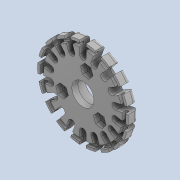
# Autodesk Inventor part: PartA
Saved by Autodesk Inventor 2020.4 (Build 244396000, 396)
## iProperties
Created: 2020-04-29
Part Number: PartA
Material: ABS Plastic
Document SubType Name: Modeling
Designer: Acer
Density: 1.06 g/cm^3
Appearance: Smooth - Black
Author: Acer
Autodesk Inventor part; units mm, degrees
ref_plane "YZ Plane" through (0, 0, 0) normal (1, 0, 0) x (0, 1, 0)
ref_plane "XZ Plane" through (0, 0, 0) normal (0, 1, 0) x (-1, 0, 0)
ref_plane "XY Plane" through (0, 0, 0) normal (0, 0, 1) x (1, 0, 0)
sketch "Sketch1" plane through (0, 0, 0) normal (0, 0, 1) x (1, 0, 0)
  circle A0 centre (0, 0) radius 22.5
  dimension "d0" = 45
  constraints: 1 centre point, 1 coincident
  measures "d0" diameter of A0
extrude "PartA Base" add sketch "Sketch1" along normal blind 7
sketch "Sketch2" plane through (0, 0, 0) normal (0, 0, -1) x (-1, 0, 0)
  circle A0 centre (0, 0) radius 13.5
  circle A1 centre (0, 0) radius 22.5 projected
  dimension "d3" = 27
  constraints: 1 centre point, 1 coincident
  measures "d3" diameter of A0
extrude "Shaft Entrance" cut sketch "Sketch2" against normal blind 2
sketch "Sketch3" plane through (0, 0, 7) normal (0, 0, 1) x (1, 0, 0)
  line L0 (0, 22.95) -> (0, 16.25) construction
  line L1 (-1.6, 22.95) -> (-1.6, 16.25)
  line L2 (1.6, 16.25) -> (1.6, 22.95)
  arc A0 (1.6, 22.95) -> (-1.6, 22.95) centre (0, 22.95) ccw
  arc A1 (-1.6, 16.25) -> (1.6, 16.25) centre (0, 16.25) ccw
  line L3 (0, 22.95) -> (6.7, 22.95) construction
  line L4 (-4.0543, 15.8172) -> (-6.3459, 22.1132)
  arc A2 (-7.0613, 14.7228) -> (-4.0543, 15.8172) centre (-5.5578, 15.27) ccw
  line L5 (-7.8494, 21.5659) -> (-5.5578, 15.27) construction
  arc A3 (-6.3459, 22.1132) -> (-9.3529, 21.0187) centre (-7.8494, 21.5659) ccw
  line L6 (-9.3529, 21.0187) -> (-7.0613, 14.7228)
  line L7 (-7.8494, 21.5659) -> (-1.5534, 23.8575) construction
  line L8 (-9.2196, 13.4767) -> (-13.5263, 18.6092)
  arc A4 (-11.671, 11.4198) -> (-9.2196, 13.4767) centre (-10.4453, 12.4482) ccw
  line L9 (-14.752, 17.5807) -> (-10.4453, 12.4482) construction
  arc A5 (-13.5263, 18.6092) -> (-15.9776, 16.5523) centre (-14.752, 17.5807) ccw
  line L10 (-15.9776, 16.5523) -> (-11.671, 11.4198)
  line L11 (-14.752, 17.5807) -> (-9.6195, 21.8874) construction
  line L12 (-13.2729, 9.5106) -> (-19.0753, 12.8606)
  arc A6 (-14.8729, 6.7394) -> (-13.2729, 9.5106) centre (-14.0729, 8.125) ccw
  line L13 (-19.8753, 11.475) -> (-14.0729, 8.125) construction
  arc A7 (-19.0753, 12.8606) -> (-20.6753, 10.0894) centre (-19.8753, 11.475) ccw
  line L14 (-20.6753, 10.0894) -> (-14.8729, 6.7394)
  line L15 (-19.8753, 11.475) -> (-16.5253, 17.2774) construction
  line L16 (-15.7253, 4.3975) -> (-22.3235, 5.5609)
  arc A8 (-16.281, 1.2461) -> (-15.7253, 4.3975) centre (-16.0031, 2.8218) ccw
  line L17 (-22.6013, 3.9852) -> (-16.0031, 2.8218) construction
  arc A9 (-22.3235, 5.5609) -> (-22.8792, 2.4095) centre (-22.6013, 3.9852) ccw
  line L18 (-22.8792, 2.4095) -> (-16.281, 1.2461)
  line L19 (-22.6013, 3.9852) -> (-21.4379, 10.5834) construction
  line L20 (-16.281, -1.2461) -> (-22.8792, -2.4095)
  arc A10 (-15.7253, -4.3975) -> (-16.281, -1.2461) centre (-16.0031, -2.8218) ccw
  line L21 (-22.6013, -3.9852) -> (-16.0031, -2.8218) construction
  arc A11 (-22.8792, -2.4095) -> (-22.3235, -5.5609) centre (-22.6013, -3.9852) ccw
  line L22 (-22.3235, -5.5609) -> (-15.7253, -4.3975)
  line L23 (-22.6013, -3.9852) -> (-23.7648, 2.613) construction
  line L24 (-14.8729, -6.7394) -> (-20.6753, -10.0894)
  arc A12 (-13.2729, -9.5106) -> (-14.8729, -6.7394) centre (-14.0729, -8.125) ccw
  line L25 (-19.8753, -11.475) -> (-14.0729, -8.125) construction
  arc A13 (-20.6753, -10.0894) -> (-19.0753, -12.8606) centre (-19.8753, -11.475) ccw
  line L26 (-19.0753, -12.8606) -> (-13.2729, -9.5106)
  line L27 (-19.8753, -11.475) -> (-23.2253, -5.6726) construction
  line L28 (-11.671, -11.4198) -> (-15.9776, -16.5523)
  arc A14 (-9.2196, -13.4767) -> (-11.671, -11.4198) centre (-10.4453, -12.4482) ccw
  line L29 (-14.752, -17.5807) -> (-10.4453, -12.4482) construction
  arc A15 (-15.9776, -16.5523) -> (-13.5263, -18.6092) centre (-14.752, -17.5807) ccw
  line L30 (-13.5263, -18.6092) -> (-9.2196, -13.4767)
  line L31 (-14.752, -17.5807) -> (-19.8845, -13.274) construction
  line L32 (-7.0613, -14.7228) -> (-9.3529, -21.0187)
  arc A16 (-4.0543, -15.8172) -> (-7.0613, -14.7228) centre (-5.5578, -15.27) ccw
  line L33 (-7.8494, -21.5659) -> (-5.5578, -15.27) construction
  arc A17 (-9.3529, -21.0187) -> (-6.3459, -22.1132) centre (-7.8494, -21.5659) ccw
  line L34 (-6.3459, -22.1132) -> (-4.0543, -15.8172)
  line L35 (-7.8494, -21.5659) -> (-14.1453, -19.2744) construction
  line L36 (-1.6, -16.25) -> (-1.6, -22.95)
  arc A18 (1.6, -16.25) -> (-1.6, -16.25) centre (0, -16.25) ccw
  line L37 (0, -22.95) -> (0, -16.25) construction
  arc A19 (-1.6, -22.95) -> (1.6, -22.95) centre (0, -22.95) ccw
  line L38 (1.6, -22.95) -> (1.6, -16.25)
  line L39 (0, -22.95) -> (-6.7, -22.95) construction
  line L40 (4.0543, -15.8172) -> (6.3459, -22.1132)
  arc A20 (7.0613, -14.7228) -> (4.0543, -15.8172) centre (5.5578, -15.27) ccw
  line L41 (7.8494, -21.5659) -> (5.5578, -15.27) construction
  arc A21 (6.3459, -22.1132) -> (9.3529, -21.0187) centre (7.8494, -21.5659) ccw
  line L42 (9.3529, -21.0187) -> (7.0613, -14.7228)
  line L43 (7.8494, -21.5659) -> (1.5534, -23.8575) construction
  line L44 (9.2196, -13.4767) -> (13.5263, -18.6092)
  arc A22 (11.671, -11.4198) -> (9.2196, -13.4767) centre (10.4453, -12.4482) ccw
  line L45 (14.752, -17.5807) -> (10.4453, -12.4482) construction
  arc A23 (13.5263, -18.6092) -> (15.9776, -16.5523) centre (14.752, -17.5807) ccw
  line L46 (15.9776, -16.5523) -> (11.671, -11.4198)
  line L47 (14.752, -17.5807) -> (9.6195, -21.8874) construction
  line L48 (13.2729, -9.5106) -> (19.0753, -12.8606)
  arc A24 (14.8729, -6.7394) -> (13.2729, -9.5106) centre (14.0729, -8.125) ccw
  line L49 (19.8753, -11.475) -> (14.0729, -8.125) construction
  arc A25 (19.0753, -12.8606) -> (20.6753, -10.0894) centre (19.8753, -11.475) ccw
  line L50 (20.6753, -10.0894) -> (14.8729, -6.7394)
  line L51 (19.8753, -11.475) -> (16.5253, -17.2774) construction
  line L52 (15.7253, -4.3975) -> (22.3235, -5.5609)
  arc A26 (16.281, -1.2461) -> (15.7253, -4.3975) centre (16.0031, -2.8218) ccw
  line L53 (22.6013, -3.9852) -> (16.0031, -2.8218) construction
  arc A27 (22.3235, -5.5609) -> (22.8792, -2.4095) centre (22.6013, -3.9852) ccw
  line L54 (22.8792, -2.4095) -> (16.281, -1.2461)
  line L55 (22.6013, -3.9852) -> (21.4379, -10.5834) construction
  line L56 (16.281, 1.2461) -> (22.8792, 2.4095)
  arc A28 (15.7253, 4.3975) -> (16.281, 1.2461) centre (16.0031, 2.8218) ccw
  line L57 (22.6013, 3.9852) -> (16.0031, 2.8218) construction
  arc A29 (22.8792, 2.4095) -> (22.3235, 5.5609) centre (22.6013, 3.9852) ccw
  line L58 (22.3235, 5.5609) -> (15.7253, 4.3975)
  line L59 (22.6013, 3.9852) -> (23.7648, -2.613) construction
  line L60 (14.8729, 6.7394) -> (20.6753, 10.0894)
  arc A30 (13.2729, 9.5106) -> (14.8729, 6.7394) centre (14.0729, 8.125) ccw
  line L61 (19.8753, 11.475) -> (14.0729, 8.125) construction
  arc A31 (20.6753, 10.0894) -> (19.0753, 12.8606) centre (19.8753, 11.475) ccw
  line L62 (19.0753, 12.8606) -> (13.2729, 9.5106)
  line L63 (19.8753, 11.475) -> (23.2253, 5.6726) construction
  line L64 (11.671, 11.4198) -> (15.9776, 16.5523)
  arc A32 (9.2196, 13.4767) -> (11.671, 11.4198) centre (10.4453, 12.4482) ccw
  line L65 (14.752, 17.5807) -> (10.4453, 12.4482) construction
  arc A33 (15.9776, 16.5523) -> (13.5263, 18.6092) centre (14.752, 17.5807) ccw
  line L66 (13.5263, 18.6092) -> (9.2196, 13.4767)
  line L67 (14.752, 17.5807) -> (19.8845, 13.274) construction
  line L68 (7.0613, 14.7228) -> (9.3529, 21.0187)
  arc A34 (4.0543, 15.8172) -> (7.0613, 14.7228) centre (5.5578, 15.27) ccw
  line L69 (7.8494, 21.5659) -> (5.5578, 15.27) construction
  arc A35 (9.3529, 21.0187) -> (6.3459, 22.1132) centre (7.8494, 21.5659) ccw
  line L70 (6.3459, 22.1132) -> (4.0543, 15.8172)
  line L71 (7.8494, 21.5659) -> (14.1453, 19.2744) construction
  point P0 (0, 0)
  point P1 (0, 19.6)
  dimension "d6" = 6.7
  dimension "d7" = 90
  dimension "d8" = 3.2
  dimension "d9" = 0
  dimension "d10" = 19.6
  dimension "d15" = 360
  constraints: 180 end point, 72 point on circle, 36 centre point, 4 tangent, 1 horizontal, 1 midpoint, 1 parallel, 1 perpendicular, 1 vertical, 235 other
  measures "d6" distance of L0.start L0.end
  measures "d7" angle of L0 L3
  measures "d8" diameter of A1
  measures "d9" horizontal distance of point (0, 0) L0.end
  measures "d10" distance of point (0, 0) point (0, 19.6)
extrude "Roller Entrance" cut sketch "Sketch3" against normal up to surface (5 mm away)
sketch "Sketch4" plane through (0, 0, 7) normal (0, 0, 1) x (1, 0, 0)
  circle A0 centre (0, 0) radius 20.4
  circle A1 centre (0, 0) radius 19.54
  circle A2 centre (0, 0) radius 21.26
  dimension "d17" = 40.8
  dimension "d18" = 39.08
  dimension "d19" = 42.52
  constraints: 3 centre point, 3 coincident
  measures "d17" diameter of A0
  measures "d18" diameter of A1
  measures "d19" diameter of A2
extrude "Wire Entrance" cut sketch "Sketch4" against normal blind 2.1 contours A0 | A2
sketch "Sketch5" plane through (0, 0, 7) normal (0, 0, 1) x (1, 0, 0)
  point P0 (0, 0)
hole "Bearing Fit" at (0, 0, 7) direction (0, 0, -1) diameter 11 depth 3
sketch "Sketch6" plane through (0, 0, 0) normal (0, 0, -1) x (-1, 0, 0)
  circle A0 centre (0, 0) radius 13.5 projected
  circle A1 centre (-1.9101, 10.833) radius 1.5
  circle A2 centre (-8.4266, -7.0707) radius 1.5
  circle A3 centre (10.3367, -3.7623) radius 1.5
  circle A4 centre (0, 0) radius 6
  dimension "d29" = 3
  dimension "d30" = 1.9101
  dimension "d31" = 10.833
  dimension "d34" = 360
  dimension "d36" = 12
  constraints: 4 centre point, 1 coincident, 7 other
  measures "d29" diameter of A1
  measures "d30" horizontal distance of A1.centre point (0, 0)
  measures "d31" vertical distance of point (0, 0) A1.centre
  measures "d36" diameter of A4
extrude "Threads and Gear Fit" cut sketch "Sketch6" against normal up to surface (7 mm away) contours A1 | A2 | A3
sketch "Sketch7" plane through (0, 0, 7) normal (0, 0, 1) x (1, 0, 0)
  circle A0 centre (-10.3367, -3.7623) radius 1.5 projected
  circle A1 centre (1.9101, 10.833) radius 1.5 projected
  circle A2 centre (8.4266, -7.0707) radius 1.5 projected
  line L0 (0, 0) -> (-10.3367, -3.7623) construction
  line L1 (0, 0) -> (1.9101, 10.833) construction
  line L2 (0, 0) -> (8.4266, -7.0707) construction
  line L3 (-7.1982, -4.3157) -> (-9.2467, -6.7571)
  line L4 (-9.2467, -6.7571) -> (-12.3853, -6.2036)
  line L5 (-12.3853, -6.2036) -> (-13.4753, -3.2089)
  line L6 (-13.4753, -3.2089) -> (-11.4267, -0.7675)
  line L7 (-11.4267, -0.7675) -> (-8.2882, -1.3209)
  line L8 (-8.2882, -1.3209) -> (-7.1982, -4.3157)
  line L9 (7.3366, -4.0759) -> (10.4751, -4.6294)
  line L10 (10.4751, -4.6294) -> (11.5651, -7.6241)
  line L11 (11.5651, -7.6241) -> (9.5166, -10.0655)
  line L12 (9.5166, -10.0655) -> (6.378, -9.5121)
  line L13 (6.378, -9.5121) -> (5.288, -6.5173)
  line L14 (5.288, -6.5173) -> (7.3366, -4.0759)
  line L15 (-0.1384, 8.3916) -> (-1.2284, 11.3864)
  line L16 (-1.2284, 11.3864) -> (0.8201, 13.8278)
  line L17 (0.8201, 13.8278) -> (3.9587, 13.2744)
  line L18 (3.9587, 13.2744) -> (5.0487, 10.2796)
  line L19 (5.0487, 10.2796) -> (3.0001, 7.8382)
  line L20 (3.0001, 7.8382) -> (-0.1384, 8.3916)
  point P0 (-7.7432, -2.8183)
  point P1 (6.3123, -5.2966)
  point P2 (1.4309, 8.1149)
  dimension "d39" = 2.76
  dimension "d40" = 2.76
  dimension "d41" = 2.76
  constraints: 42 end point, 3 coincident, 3 midpoint, 3 point on line, 39 other
  measures "d39" distance from line of L14 L2.end
  measures "d40" distance from line of L20 L1.end
  measures "d41" distance from line of L8 L0.end
extrude "M3 Nut" cut sketch "Sketch7" against normal blind 2.55 contours A0 | A1 | A2 | L3 L4 L5 L6 L7 L8 | L9 L10 L11 L12 L13 L14 | L15 L16 L17 L18 L19 L20
fillet "Wire and Ground Rounding" radius 2 18 edges at (11.25, -19.4856, 2) (3.9071, -22.1582, 2) (-3.9071, -22.1582, 2) (-11.25, -19.4856, 2) (-17.236, -14.4627, 2) (-21.1431, -7.6955, 2) (-22.5, 0, 2) (-21.1431, 7.6955, 2) (-17.236, 14.4627, 2) (-11.25, 19.4856, 2) (-3.9071, 22.1582, 2) (3.9071, 22.1582, 2) (11.25, 19.4856, 2) (17.236, 14.4627, 2) (21.1431, 7.6955, 2) (22.5, 0, 2) (21.1431, -7.6955, 2) (17.236, -14.4627, 2)
fillet "Wire and Ground Rounding" radius 0.625 36 edges at (-19.9779, -7.2713, 4.9) (-16.2861, -13.6657, 4.9) (-10.63, -18.4117, 4.9) (-3.6918, -20.937, 4.9) (3.6918, -20.937, 4.9) (10.63, -18.4117, 4.9) (16.2861, -13.6657, 4.9) (19.9779, -7.2713, 4.9) (21.26, 0, 4.9) (19.9779, 7.2713, 4.9) (16.2861, 13.6657, 4.9) (10.63, 18.4117, 4.9) (3.6918, 20.937, 4.9) (-3.6918, 20.937, 4.9) (-10.63, 18.4117, 4.9) (-16.2861, 13.6657, 4.9) (-19.9779, 7.2713, 4.9) (-21.26, 0, 4.9) (-19.54, 0, 4.9) (-18.3616, -6.6831, 4.9) (-14.9685, -12.5601, 4.9) (-9.77, -16.9221, 4.9) (-3.3931, -19.2431, 4.9) (3.3931, -19.2431, 4.9) (9.77, -16.9221, 4.9) (14.9685, -12.5601, 4.9) (18.3616, -6.6831, 4.9) (19.54, 0, 4.9) (18.3616, 6.6831, 4.9) (14.9685, 12.5601, 4.9) (9.77, 16.9221, 4.9) (3.3931, 19.2431, 4.9) (-3.3931, 19.2431, 4.9) (-18.3616, 6.6831, 4.9) (-14.9685, 12.5601, 4.9) (-9.77, 16.9221, 4.9)
sketch "Sketch8" plane through (0, 0, 0) normal (0, 0, -1) x (-1, 0, 0)
  circle A0 centre (0, 0) radius 5.5 projected
  circle A1 centre (0, 0) radius 6
  dimension "d46" = 12
  constraints: 1 centre point, 1 coincident
  measures "d46" diameter of A1
extrude "Extrusion7" cut sketch "Sketch8" against normal up to surface (4 mm away) contours A0 | A1
body "Solid1"
